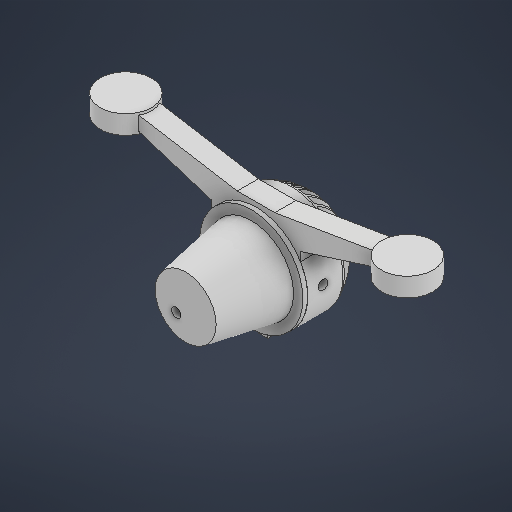
# Autodesk Inventor part: Diff V2
Saved by Autodesk Inventor 2026.1 (Build 301233000, 233)
## iProperties
Created: 2026-08-04
Part Number: Diff V2
Material: Generic
Document SubType Name: Modeling
Designer: share
Density: 1 g/cm^3
Appearance: Default
Author: share
Autodesk Inventor part; units mm, degrees
ref_plane "XZ Plane" through (0, 0, 0) normal (0, 1, 0) x (-1, 0, 0)
sketch "Sketch3" plane through (0, 0, 0) normal (0, 0, 1) x (1, 0, 0)
  circle A0 centre (0, 0) radius 65
  dimension "d8" = 130
  constraints: 1 centre point, 1 coincident
  measures "d8" diameter of A0
ref_plane "Front Section Flange Plane" through (0, 0, -140) normal (0, 0, 1) x (1, 0, 0)
sketch "Sketch4" plane through (0, 0, -140) normal (0, 0, 1) x (1, 0, 0)
  circle A0 centre (0, 0) radius 90
  dimension "d13" = 180
  constraints: 1 centre point, 1 coincident
  measures "d13" diameter of A0
loft "Main Body" add profiles "Sketch3", "Sketch4"
sketch "Sketch5" plane through (0, 0, -140) normal (0, 0, 1) x (1, 0, 0)
  circle A0 centre (0, 0) radius 90 projected
  circle A1 centre (0, 0) radius 110
  dimension "d18" = 20
  constraints: 1 centre point, 1 coincident
  measures "d18" radial gap between concentric circles of A1 A0
extrude "Front Flange" add sketch "Sketch5" against normal blind 10 contours A0 | A1
sketch "Sketch6" plane through (0, 0, -150) normal (0, 0, -1) x (-1, 0, 0)
  circle A0 centre (0, 0) radius 110.5
  dimension "d21" = 221
  constraints: 1 centre point, 1 coincident
  measures "d21" diameter of A0
extrude "MidSection" add sketch "Sketch6" along normal blind 45
sketch "Sketch7" plane through (0, 0, -195) normal (0, 0, -1) x (-1, 0, 0)
  line L0 (0, -176.5) -> (0, 215.5) construction
  line L1 (-490, 0) -> (490, 0) construction
  line L2 (-40, 119.5) -> (40, 119.5)
  circle A0 centre (0, 0) radius 110.5 projected
  line L3 (0, 0) -> (0, 110) construction
  circle A1 centre (0, 0) radius 110 projected
  line L4 (-40, 119.5) -> (-250, 154.5)
  line L5 (-250, 154.5) -> (-250, 159.5)
  line L6 (-250, 159.5) -> (-350, 159.5)
  line L7 (-350, 159.5) -> (-350, 119.5)
  line L8 (-350, 119.5) -> (-250, 119.5)
  line L9 (-250, 119.5) -> (-250, 124.5)
  line L10 (-250, 124.5) -> (-95, 75.4527)
  line L11 (-95, 75.4527) -> (-95, 55.4527)
  line L12 (40, 119.5) -> (250, 154.5)
  line L13 (250, 154.5) -> (250, 159.5)
  line L14 (250, 159.5) -> (350, 159.5)
  line L15 (350, 159.5) -> (350, 119.5)
  line L16 (350, 119.5) -> (250, 119.5)
  line L17 (250, 119.5) -> (250, 124.5)
  line L18 (250, 124.5) -> (95, 75.4527)
  line L19 (95, 75.4527) -> (95, 55.4527)
  line L20 (-250, 154.5) -> (-250, 124.5) construction
  line L21 (250, 154.5) -> (250, 124.5) construction
  line L22 (-350, 139.5) -> (-250, 139.5) construction
  line L23 (-25, -110.5) -> (25, -110.5) construction
  line L24 (-25, -110.5) -> (-25, -120.5)
  line L25 (-25, -120.5) -> (-5, -120.5)
  line L26 (-5, -120.5) -> (-5, -110.3868)
  line L27 (25, -110.5) -> (25, -120.5)
  line L28 (25, -120.5) -> (5, -120.5)
  line L29 (5, -120.5) -> (5, -110.3868)
  line L30 (-25, -110.5) -> (-25, -107.6348)
  line L31 (25, -110.5) -> (25, -107.6348)
  point P0 (0, 119.5)
  point P1 (0, -110.5)
  point P2 (-5, -110.5)
  point P3 (5, -110.5)
  point P4 (-95, 56.438)
  point P5 (95, 56.438)
  dimension "d25" = 80
  dimension "d26" = 700
  dimension "d27" = 40
  dimension "d28" = 5
  dimension "d29" = 100
  dimension "d35" = 50
  dimension "d37" = 10
  dimension "d38" = 20
  dimension "d41" = 240
  dimension "d42" = 280
  dimension "d44" = 20
  dimension "d73" = 190
  constraints: 60 end point, 11 symmetric about line, 10 point on line, 8 perpendicular, 7 point on circle, 4 midpoint, 4 vertical, 2 collinear, 1 parallel, 1 tangent
  measures "d25" distance of L2.start L2.end
  measures "d26" distance between parallel lines of L15 L7
  measures "d27" distance between parallel lines of L8 L6
  measures "d28" distance of L4.end L5.end
  measures "d29" distance between parallel lines of L20 L7
  measures "d35" distance of L23.start L23.end
  measures "d37" distance between parallel lines of L25 L23
  measures "d38" distance between parallel lines of L26 L24
  measures "d41" distance between parallel lines of L25 L2
  measures "d42" distance between parallel lines of L6 L25
  measures "d44" distance of L10.end L11.end
  measures "d73" distance between parallel lines of L19 L11
extrude "T Mount" add sketch "Sketch7" against normal up to surface (45 mm away) contours L2 L12 L13 L14 L15 L16 L17 L18 L19 A0 L11 L10 L9 L8 L7 L6 L5 L4 | A0 L26 L25 L24 L30 | L31 L27 L28 L29 A0
sketch "Sketch9" plane through (0, 0, 0) normal (1, 0, 0) x (0, 1, 0)
  line L0 (0, 39) -> (0, -234) construction
  line L1 (-110.5, -150) -> (-110.5, -195) construction
  line L2 (-110.5, -195) -> (-110.3868, -195) projected
  line L3 (-110.3868, -195) -> (0, -195)
  line L4 (-110.5, -195) -> (-110.5, -225)
  line L5 (110.3868, -195) -> (0, -195)
  line L6 (110.5, -195) -> (110.5, -225)
  arc A0 (-110.5, -225) -> (110.5, -225) centre (0, -181.0983) ccw
  line L7 (0, -195) -> (0, -300)
  line L8 (-107.6348, -150) -> (56.438, -150) projected
  line L9 (-107.6348, -150) -> (-120.5, -150) projected
  line L10 (-120.5, -150) -> (-110.3868, -150) projected
  line L11 (-110.3868, -150) -> (-110.3868, -150) projected
  line L12 (-110.3868, -150) -> (-120.5, -150) projected
  line L13 (-120.5, -150) -> (-107.6348, -150) projected
  line L14 (56.438, -150) -> (-107.6348, -150) projected
  line L15 (56.438, -150) -> (75.4527, -150) projected
  line L16 (75.4527, -150) -> (124.5, -150) projected
  line L17 (124.5, -150) -> (119.5, -150) projected
  line L18 (119.5, -150) -> (159.5, -150) projected
  line L19 (159.5, -150) -> (154.5, -150) projected
  line L20 (154.5, -150) -> (119.5, -150) projected
  line L21 (119.5, -150) -> (154.5, -150) projected
  line L22 (154.5, -150) -> (159.5, -150) projected
  line L23 (159.5, -150) -> (119.5, -150) projected
  line L24 (119.5, -150) -> (124.5, -150) projected
  line L25 (124.5, -150) -> (75.4527, -150) projected
  line L26 (75.4527, -150) -> (56.438, -150) projected
  line L27 (-110, -150) -> (110, -150) projected
  point P0 (0, 0)
  dimension "d56" = 30
  dimension "d59" = 150
  constraints: 10 end point, 3 point on circle, 3 symmetric about line, 1 centre point, 1 parallel, 1 perpendicular, 1 point on line
  measures "d56" distance of L1.end L4.end
  measures "d59" distance from line of L7.end L20
revolve "Rear Section" add sketch "Sketch9" angle 360 about axis through (0, 0, -195) along (0, 0, -1)
sketch "Sketch10" plane through (0, 0, 0) normal (0, 0, 1) x (1, 0, 0)
  line L0 (0, 215.5) -> (0, -176.5) construction
  line L1 (-490, 0) -> (490, 0) construction
  circle A0 centre (-20, -20) radius 10
  point P0 (0, 0)
  dimension "d61" = 20
  dimension "d62" = 20
  dimension "d63" = 20
  constraints: 1 centre point
  measures "d61" distance from line of A0.centre L1
  measures "d62" distance from line of A0.centre L0
  measures "d63" diameter of A0
extrude "Front Flange Hole" cut sketch "Sketch10" against normal blind 20
ref_plane "CV Flange Plane" through (110.5, 0, -150) normal (1, 0, 0) x (0, 1, 0)
sketch "Sketch11" plane through (110.5, 0, -150) normal (1, 0, 0) x (0, 1, 0)
  line L0 (-110.5, 0) -> (-110.5, -75) projected
  line L1 (110.5, -45) -> (110.5, -75) projected
  line L2 (110, 10) -> (-110, 10) projected
  line L3 (-110.5, -75) -> (110.5, -75) projected
  line L4 (-110, 10) -> (-110.5, 10)
  line L5 (-110.5, 0) -> (-110.5, 10)
  line L6 (-110.5, 10) -> (-110.5, -75)
  line L7 (110, 10) -> (110.5, -45)
  line L8 (-110.5, -32.5) -> (110.3864, -32.5) construction
  line L9 (0, 10) -> (0, -75) construction
  circle A0 centre (5, -32.5) radius 10
  point P0 (0, 150)
  dimension "d66" = 5
  dimension "d67" = 20
  constraints: 12 end point, 3 midpoint, 2 horizontal, 2 point on line, 1 centre point, 1 collinear, 1 perpendicular
  measures "d66" distance from line of L9 A0.centre
  measures "d67" diameter of A0
extrude "CV Flange Hole" cut sketch "Sketch11" against normal through all contours A0
sketch "Sketch12" plane through (250, 159.5, -195) normal (0, 1, 0) x (1, 0, 0)
  line L0 (100, -45) -> (0, -45) construction
  line L1 (100, 0) -> (100, -45) construction
  line L2 (0, 0) -> (100, 0) construction
  line L3 (0, 0) -> (0, -45) construction
  line L4 (100, -22.5) -> (0, -22.5) construction
  line L5 (0, -45) -> (-210, -45) projected
  circle A0 centre (50, -22.5) radius 54.8293
  line L6 (-250, 77.7951) -> (-250, -240.4659) construction
  circle A1 centre (-550, -22.5) radius 54.8293
  point P0 (-250, -195)
  constraints: 3 midpoint, 2 end point, 1 centre point, 1 symmetric about line, 4 other
extrude "Mounting Pucks" add sketch "Sketch12" against normal up to surface (40 mm away)
ref_plane "Work Plane5" through (0, 0, -300) normal (0, 0, 1) x (1, 0, 0)
sketch "Sketch13" plane through (0, 0, -300) normal (0, 0, 1) x (1, 0, 0)
  circle A0 centre (0, 0) radius 110.5 projected
  line L0 (45, 100.922) -> (45, -100.922)
  line L1 (30, 106.3497) -> (30, -106.3497)
  arc A1 (95, 56.438) -> (-95, 56.438) centre (0, 0) ccw projected
  line L2 (10, 110.0466) -> (10, -110.0466)
  line L3 (5, -110.3868) -> (5, 110.3868)
  line L4 (25, 107.6348) -> (25, -107.6348)
  line L5 (0, 215.5) -> (0, -176.5) projected
  line L6 (50, 98.5406) -> (50, -98.5406)
  line L7 (70, 85.5) -> (70, -85.5)
  line L8 (65, 89.3602) -> (65, -89.3602)
  line L9 (90, 64.1112) -> (90, -64.1112)
  line L10 (85, 70.6063) -> (85, -70.6063)
  line L11 (-45, 100.922) -> (-45, -100.922)
  line L12 (-30, 106.3497) -> (-30, -106.3497)
  line L13 (-10, 110.0466) -> (-10, -110.0466)
  line L14 (-5, -110.3868) -> (-5, 110.3868)
  line L15 (-25, 107.6348) -> (-25, -107.6348)
  line L16 (-50, 98.5406) -> (-50, -98.5406)
  line L17 (-70, 85.5) -> (-70, -85.5)
  line L18 (-65, 89.3602) -> (-65, -89.3602)
  line L19 (-90, 64.1112) -> (-90, -64.1112)
  line L20 (-85, 70.6063) -> (-85, -70.6063)
  point P0 (-70, -85.5)
  dimension "d76" = 5
  dimension "d77" = 5
  dimension "d78" = 10
  dimension "d79" = 30
  dimension "d81" = 5
  dimension "d82" = 50
  dimension "d83" = 5
  dimension "d84" = 70
  dimension "d85" = 5
  dimension "d86" = 90
  constraints: 40 end point, 20 symmetric about line, 4 parallel, 4 vertical, 22 other
  measures "d76" distance between parallel lines of L3 L2
  measures "d77" distance between parallel lines of L4 L1
  measures "d78" distance between parallel lines of L2 L5
  measures "d79" distance between parallel lines of L1 L5
  measures "d81" distance between parallel lines of L0 L6
  measures "d82" distance between parallel lines of L5 L6
  measures "d83" distance between parallel lines of L8 L7
  measures "d84" distance between parallel lines of L5 L7
  measures "d85" distance between parallel lines of L10 L9
  measures "d86" distance between parallel lines of L5 L9
extrude "Extrusion7" cut sketch "Sketch13" along normal blind 70 contours A0 L9 | A0 L7 L10 | A0 L6 L8 | A0 L1 L0 | A0 L2 L4 | A0 L5 L3 | A0 L14 L5 | A0 L15 L13 | A0 L11 L12 | A0 L18 L16 | A0 L20 L17 | A0 L19
body "Solid2"
